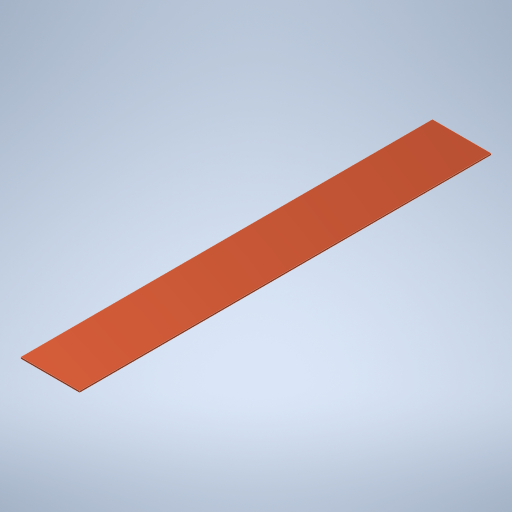
# Autodesk Inventor part: Pigtail
Saved by Autodesk Inventor 2023 (Build 270158000, 158)
## iProperties
Created: 2023-03-15
Part Number: Pigtail
Material: Copper
Document SubType Name: Modeling
Designer: Caleb
Density: 8.94 g/cm^3
Appearance: Copper - Satin
Author: Caleb
Autodesk Inventor part; units mm, degrees
ref_plane "YZ Plane" through (0, 0, 0) normal (1, 0, 0) x (0, 1, 0)
ref_plane "XZ Plane" through (0, 0, 0) normal (0, 1, 0) x (-1, 0, 0)
ref_plane "XY Plane" through (0, 0, 0) normal (0, 0, 1) x (1, 0, 0)
sketch "Sketch1" plane through (0, 0, 0) normal (0, 1, 0) x (-1, 0, 0)
  line L0 (-5, -35) -> (5, -35)
  line L1 (5, -35) -> (5, 35)
  line L2 (5, 35) -> (-5, 35)
  line L3 (-5, 35) -> (-5, -35)
  line L4 (-5, -35) -> (5, 35) construction
  line L5 (5, -35) -> (-5, 35) construction
  point P0 (0, 0)
  dimension "d0" = 70
  dimension "d1" = 10
  constraints: 12 end point, 2 midpoint, 2 parallel, 1 horizontal, 1 perpendicular
  measures "d0" distance of L0.end L1.end
  measures "d1" distance of L1.end L2.end
extrude "Extrusion1" add sketch "Sketch1" along normal blind 0.254
body "Solid1"
